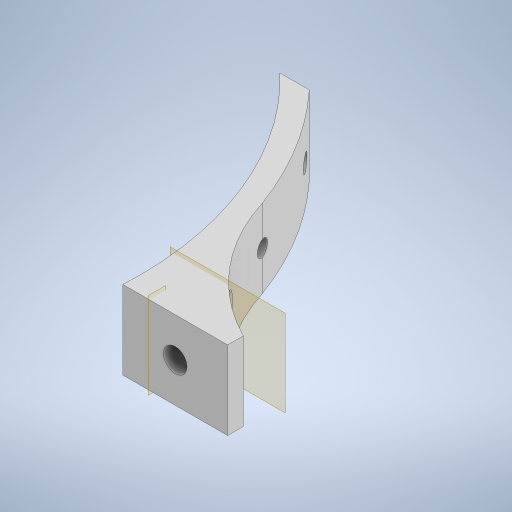
# Autodesk Inventor part: armGuide
Saved by Autodesk Inventor 2024.2 (Build 282272000, 272)
## iProperties
Created: 2024-06-04
Part Number: armGuide
Material: Generic
Document SubType Name: Modeling
Designer: Robin
Density: 1 g/cm^3
Appearance: Default
Author: Robin
Autodesk Inventor part; units mm, degrees
ref_plane "YZ Plane" through (0, 0, 0) normal (1, 0, 0) x (0, 1, 0)
ref_plane "XZ Plane" through (0, 0, 0) normal (0, 1, 0) x (-1, 0, 0)
ref_plane "XY Plane" through (0, 0, 0) normal (0, 0, 1) x (1, 0, 0)
sketch "Sketch1" plane through (0, 0, 0) normal (0, 1, 0) x (-1, 0, 0)
  line L0 (0, 0) -> (40, 0)
  line L1 (40, 0) -> (40, -50)
  line L2 (40, -50) -> (0, -50)
  line L3 (0, -50) -> (0, 0)
  arc A0 (20, 0) -> (40, -50) centre (84.9294, -3.0282) ccw
  arc A1 (16, 0) -> (34.3914, -50) centre (84.9294, -3.0282) ccw
  arc A2 (20.1752, -26.8467) -> (0, -3) centre (-18.0257, -38.7082) ccw
  point P0 (20, 0)
  dimension "d0" = 40
  dimension "d1" = 50
  dimension "d2" = 65
  dimension "d3" = 20
  dimension "d4" = 4
  dimension "d5" = 40
  dimension "d6" = 3
  constraints: 8 end point, 7 point on circle, 3 centre point, 3 point on line, 2 midpoint, 2 parallel, 1 concentric, 1 horizontal, 1 perpendicular
  measures "d0" distance of L1.end L2.end
  measures "d1" distance of L0.end L1.end
  measures "d2" radius of A0
  measures "d3" distance of L0.start A0.start
  measures "d4" distance of point (20, 0) A1.start
  measures "d5" radius of A2
  measures "d6" distance of L0.start A2.end
extrude "Extrusion1" add sketch "Sketch1" along normal blind 15 contours L0 A1 A2 L3 | L0 A0 L2 A1 A2
sketch "Sketch2" plane through (-20, 0, 0) normal (0, 0, 1) x (1, 0, 0)
  circle A0 centre (10, 7.5) radius 2.25
  line L0 (0, 0) -> (0, 15) projected
  point P0 (20, 0)
  point P1 (0, 7.5)
  point P2 (0, 7.5)
  dimension "d9" = 4.5
  dimension "d10" = 10
  constraints: 2 midpoint, 1 centre point, 1 horizontal alignment
  measures "d9" diameter of A0
  measures "d10" distance of point (0, 7.5) A0.centre
extrude "Extrusion2" cut sketch "Sketch2" against normal through all
ref_plane "Work Plane1" through (-20, 0, -10) normal (0, 0, 1) x (1, 0, 0)
sketch "Sketch3" plane through (-20, 0, -10) normal (0, 0, 1) x (1, 0, 0)
  circle A0 centre (10, 7.5) radius 2.25 projected
  circle A1 centre (10, 7.5) radius 4.5
  point P0 (20, 0)
  dimension "d14" = 9
  constraints: 1 centre point, 1 coincident
  measures "d14" diameter of A1
extrude "Extrusion3" cut sketch "Sketch3" along normal blind 6 and the other way blind 10
ref_plane "Work Plane2" through (-15, 0, 0) normal (1, 0, 0) x (0, 0, -1)
sketch "Sketch4" plane through (-15, 0, 0) normal (1, 0, 0) x (0, 0, -1)
  circle A0 centre (45, 7.5) radius 1.5
  line L0 (26.8467, 0) -> (26.8467, 15) projected
  circle A1 centre (26.8467, 7.5) radius 1.5
  line L1 (50, 0) -> (50, 15) projected
  point P0 (0, 0)
  dimension "d20" = 3
  dimension "d21" = 3
  dimension "d22" = 5
  constraints: 2 centre point, 1 horizontal alignment, 1 midpoint
  measures "d20" diameter of A0
  measures "d21" diameter of A1
  measures "d22" distance from line of L1 A0.centre
extrude "Extrusion4" cut sketch "Sketch4" against normal up to surface round surface about axis through (-84.9294, 0, -3.0282) along (0, 1, 0) radius 65 far side no
sketch "Sketch6" plane through (-15, 0, 0) normal (1, 0, 0) x (0, 0, -1)
  circle A0 centre (5, 7.5) radius 1.75
  line L0 (0, 0) -> (0, 15) projected
  point P0 (0, 7.5)
  dimension "d25" = 3.5
  dimension "d26" = 5
  constraints: 1 centre point, 1 horizontal alignment, 1 midpoint
  measures "d25" diameter of A0
  measures "d26" distance from line of L0 A0.centre
extrude "Extrusion5" cut sketch "Sketch6" against normal through all
body "Solid1"
